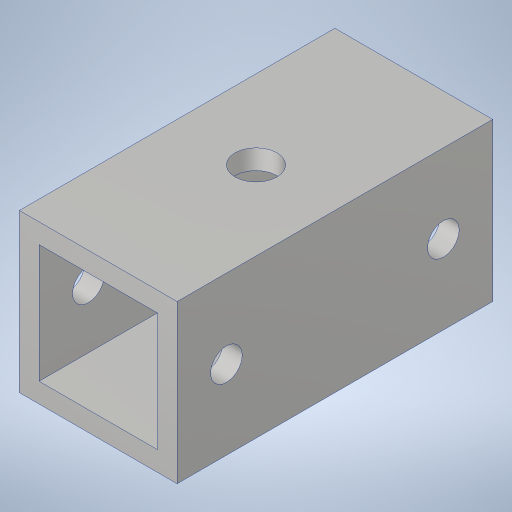
# Autodesk Inventor part: EL2-S-004
Saved by Autodesk Inventor 2023.4 (Build 274418000, 418)
## iProperties
RuleStatus: InUse
Created: 2025-01-13
Part Number: EL2-S-004
Material: Aluminum 6061
Document SubType Name: Modeling
Designer: mavericks
Mass: 304.185 g
Surface Area: 718.547 cm^2
Volume: 112.661 cm^3
Density: 2.7 g/cm^3
Appearance: Aluminum - Flat
AfterDocNew0: SHOW
AfterDocOpen0: SHOW
Author: mavericks
Autodesk Inventor part; units mm, degrees
ref_plane "YZ Plane" through (0, 0, 0) normal (1, 0, 0) x (0, 1, 0)
ref_plane "XZ Plane" through (0, 0, 0) normal (0, 1, 0) x (-1, 0, 0)
ref_plane "XY Plane" through (0, 0, 0) normal (0, 0, 1) x (1, 0, 0)
sketch "Sketch1" plane through (0, 0, 0) normal (0, 0, 1) x (1, 0, 0)
  line L0 (-12.7, -12.7) -> (12.7, -12.7)
  line L1 (12.7, -12.7) -> (12.7, 12.7)
  line L2 (12.7, 12.7) -> (-12.7, 12.7)
  line L3 (-12.7, 12.7) -> (-12.7, -12.7)
  line L4 (-12.7, -12.7) -> (12.7, 12.7) construction
  line L5 (12.7, -12.7) -> (-12.7, 12.7) construction
  line L6 (-9.525, 9.525) -> (9.525, 9.525)
  line L7 (9.525, 9.525) -> (9.525, -9.525)
  line L8 (9.525, -9.525) -> (-9.525, -9.525)
  line L9 (-9.525, -9.525) -> (-9.525, 9.525)
  point P0 (0, 0)
  dimension "width" = 25.4
  dimension "height" = 25.4
  dimension "thickness" = 3.175
  constraints: 20 end point, 4 parallel, 2 midpoint, 2 perpendicular, 1 horizontal, 3 other
  measures "width" distance of L2.end L1.end
  measures "height" distance of L1.end L0.end
  measures "thickness" distance between parallel lines of L2 L6
extrude "Extrusion1" add sketch "Sketch1" along normal mid plane 50.8
sketch "Sketch3" plane through (12.7, -12.7, 25.4) normal (1, 0, 0) x (0, 0, -1)
  line L0 (7.9375, 12.7) -> (42.8625, 12.7) construction
  point P0 (25.4, 12.7)
  point P1 (25.4, 12.7)
  dimension "d22" = 34.925
  constraints: 2 coincident, 2 end point, 2 horizontal alignment, 1 horizontal, 1 midpoint
  measures "d22" distance of L0.start L0.end
hole "Hole2" at (12.7, 0, -17.4625) at (12.7, 0, 17.4625) direction (-1, 0, 0) diameter 5.1054 end through all clearance for "Flat Head Machine Screw (82)" size "#10" standard "Ansi Unified Screw Threads"
sketch "Sketch4" plane through (-12.7, 12.7, 25.4) normal (0, 1, 0) x (1, 0, 0)
  point P0 (12.7, 25.4)
  point P1 (12.7, 25.4)
  constraints: 1 coincident
hole "Hole3" at (0, 12.7, 0) direction (0, -1, 0) diameter 6.7564 end through all clearance for "Flat Head Machine Screw (82)" size "1/4" standard "Ansi Unified Screw Threads"
body "Solid1"
